Autodesk Fusion 360 part; units mm, degrees
(part 5 of 5)
sketch "Sketch13" plane through (0, 0, 4.8) normal (0, 0, 1) x (-1, 0, 0)
  circle A0 centre (1.7941, 104.2) radius 6.1
  arc A1 (-97.4773, 89.7465) -> (-97.2023, 84.7376) centre (-94.9024, 87.3758) ccw
  line L0 (-97.2023, 84.7376) -> (-47.1809, 41.1307)
  arc A2 (-48.1666, 38.5) -> (-47.1809, 41.1307) centre (-48.1666, 40) ccw
  line L1 (-48.1666, 38.5) -> (-100, 38.5)
  arc A3 (-100, 38.5) -> (-103, 35.5) centre (-100, 35.5) ccw
  line L2 (-103, 35.5) -> (-103, 28.5)
  arc A4 (-103, 28.5) -> (-100, 25.5) centre (-100, 28.5) ccw
  line L3 (-100, 25.5) -> (-42.1213, 25.5)
  arc A5 (-40, 23.3787) -> (-42.1213, 25.5) centre (-41.0607, 24.4393) ccw
  line L4 (-40, 23.3787) -> (-40, 20.8)
  arc A6 (-40, 20.8) -> (-37.5, 18.3) centre (-37.5, 20.8) ccw
  line L5 (-37.5, 18.3) -> (-34.1213, 18.3)
  arc A7 (-32, 16.1787) -> (-34.1213, 18.3) centre (-33.0607, 17.2393) ccw
  line L6 (-32, 16.1787) -> (-32, -16.1787)
  arc A8 (-34.1213, -18.3) -> (-32, -16.1787) centre (-33.0607, -17.2393) ccw
  line L7 (-34.1213, -18.3) -> (-37.5, -18.3)
  arc A9 (-37.5, -18.3) -> (-40, -20.8) centre (-37.5, -20.8) ccw
  line L8 (-40, -20.8) -> (-40, -23.3787)
  arc A10 (-42.1213, -25.5) -> (-40, -23.3787) centre (-41.0607, -24.4393) ccw
  line L9 (-42.1213, -25.5) -> (-100, -25.5)
  arc A11 (-100, -25.5) -> (-103, -28.5) centre (-100, -28.5) ccw
  line L10 (-103, -28.5) -> (-103, -35.5)
  arc A12 (-103, -35.5) -> (-100, -38.5) centre (-100, -35.5) ccw
  line L11 (-100, -38.5) -> (-48.1666, -38.5)
  arc A13 (-47.1809, -41.1307) -> (-48.1666, -38.5) centre (-48.1666, -40) ccw
  line L12 (-47.1809, -41.1307) -> (-97.2023, -84.7376)
  arc A14 (-97.2023, -84.7376) -> (-97.4773, -89.7465) centre (-94.9024, -87.3758) ccw
  arc A15 (-97.4773, -89.7465) -> (-89.0244, -98.1371) centre (0, 0) ccw
  arc A16 (-89.0244, -98.1371) -> (-85.1797, -97.5355) centre (-87.3447, -96.2855) ccw
  line L13 (-85.1797, -97.5355) -> (-74.6084, -79.2255)
  arc A17 (-71.7106, -78.449) -> (-74.6084, -79.2255) centre (-73.1595, -78.8372) ccw
  line L14 (-71.7106, -78.449) -> (-32.0836, -101.3277)
  arc A18 (-31.3071, -104.2255) -> (-32.0836, -101.3277) centre (-31.6953, -102.7766) ccw
  line L15 (-31.3071, -104.2255) -> (-41.8784, -122.5355)
  arc A19 (-41.8784, -122.5355) -> (-40.477, -126.166) centre (-39.7133, -123.7855) ccw
  arc A20 (-40.477, -126.166) -> (129.5015, -28.0288) centre (0, 0) ccw
  arc A21 (129.5015, -28.0288) -> (127.0581, -25) centre (127.0581, -27.5) ccw
  line L16 (127.0581, -25) -> (105.9155, -25)
  arc A22 (103.7941, -22.8787) -> (105.9155, -25) centre (104.8548, -23.9393) ccw
  line L17 (103.7941, -22.8787) -> (103.7941, 22.8787)
  arc A23 (105.9155, 25) -> (103.7941, 22.8787) centre (104.8548, 23.9393) ccw
  line L18 (105.9155, 25) -> (127.0581, 25)
  arc A24 (127.0581, 25) -> (129.5015, 28.0288) centre (127.0581, 27.5) ccw
  arc A25 (129.5015, 28.0288) -> (-40.477, 126.166) centre (0, 0) ccw
  arc A26 (-40.477, 126.166) -> (-41.8784, 122.5355) centre (-39.7133, 123.7855) ccw
  line L19 (-41.8784, 122.5355) -> (-31.3071, 104.2255)
  arc A27 (-32.0836, 101.3277) -> (-31.3071, 104.2255) centre (-31.6953, 102.7766) ccw
  line L20 (-32.0836, 101.3277) -> (-71.7106, 78.449)
  arc A28 (-74.6084, 79.2255) -> (-71.7106, 78.449) centre (-73.1595, 78.8372) ccw
  line L21 (-74.6084, 79.2255) -> (-85.1797, 97.5355)
  arc A29 (-85.1797, 97.5355) -> (-89.0244, 98.1371) centre (-87.3447, 96.2855) ccw
  arc A30 (-89.0244, 98.1371) -> (-97.4773, 89.7465) centre (0, 0) ccw
  circle A31 centre (-28.2185, 125.8758) radius 1.5
  arc A32 (-52.8202, -75.7299) -> (-55.718, -76.5064) centre (-54.2691, -76.1181) ccw
  line L22 (-52.8202, -75.7299) -> (-39.1739, -83.6086)
  arc A33 (-38.3975, -86.5064) -> (-39.1739, -83.6086) centre (-38.7857, -85.0575) ccw
  line L23 (-38.3975, -86.5064) -> (-38.6762, -86.9891)
  arc A34 (-41.5739, -87.7655) -> (-38.6762, -86.9891) centre (-40.125, -87.3773) ccw
  line L24 (-41.5739, -87.7655) -> (-55.2202, -79.8868)
  arc A35 (-55.9967, -76.9891) -> (-55.2202, -79.8868) centre (-55.6084, -78.438) ccw
  line L25 (-55.9967, -76.9891) -> (-55.718, -76.5064)
  circle A36 centre (123.1209, -38.5) radius 1.5
  arc A37 (-11.2762, 39.5309) -> (-14.1739, 40.3073) centre (-12.725, 39.9191) ccw
  line L26 (-11.2762, 39.5309) -> (-10.9975, 39.0482)
  arc A38 (-11.7739, 36.1504) -> (-10.9975, 39.0482) centre (-11.3857, 37.5993) ccw
  line L27 (-11.7739, 36.1504) -> (-25.4202, 28.2717)
  arc A39 (-28.318, 29.0482) -> (-25.4202, 28.2717) centre (-26.8691, 28.66) ccw
  line L28 (-28.318, 29.0482) -> (-28.5967, 29.5309)
  arc A40 (-27.8202, 32.4286) -> (-28.5967, 29.5309) centre (-28.2084, 30.9798) ccw
  line L29 (-27.8202, 32.4286) -> (-14.1739, 40.3073)
  arc A41 (-10.9975, -39.0482) -> (-11.7739, -36.1504) centre (-11.3857, -37.5993) ccw
  line L30 (-10.9975, -39.0482) -> (-11.2762, -39.5309)
  arc A42 (-14.1739, -40.3073) -> (-11.2762, -39.5309) centre (-12.725, -39.9191) ccw
  line L31 (-14.1739, -40.3073) -> (-27.8202, -32.4286)
  arc A43 (-28.5967, -29.5309) -> (-27.8202, -32.4286) centre (-28.2084, -30.9798) ccw
  line L32 (-28.5967, -29.5309) -> (-28.318, -29.0482)
  arc A44 (-25.4202, -28.2717) -> (-28.318, -29.0482) centre (-26.8691, -28.66) ccw
  line L33 (-25.4202, -28.2717) -> (-11.7739, -36.1504)
  circle A45 centre (64.5, -111.7173) radius 1.5
  arc A46 (39.8728, -10) -> (41.9941, -7.8787) centre (40.9335, -8.9393) ccw
  line L34 (39.8728, -10) -> (39.3155, -10)
  arc A47 (37.1941, -7.8787) -> (39.3155, -10) centre (38.2548, -8.9393) ccw
  line L35 (37.1941, -7.8787) -> (37.1941, 7.8787)
  arc A48 (39.3155, 10) -> (37.1941, 7.8787) centre (38.2548, 8.9393) ccw
  line L36 (39.3155, 10) -> (39.8728, 10)
  arc A49 (41.9941, 7.8787) -> (39.8728, 10) centre (40.9335, 8.9393) ccw
  line L37 (41.9941, 7.8787) -> (41.9941, -7.8787)
  circle A50 centre (-94.9024, -87.3758) radius 1.5
  circle A51 centre (-28.2185, -125.8758) radius 1.5
  circle A52 centre (64.5, 111.7173) radius 1.5
  arc A53 (-55.2202, 79.8868) -> (-55.9967, 76.9891) centre (-55.6084, 78.438) ccw
  line L38 (-55.2202, 79.8868) -> (-41.5739, 87.7655)
  arc A54 (-38.6762, 86.9891) -> (-41.5739, 87.7655) centre (-40.125, 87.3773) ccw
  line L39 (-38.6762, 86.9891) -> (-38.3975, 86.5064)
  arc A55 (-39.1739, 83.6086) -> (-38.3975, 86.5064) centre (-38.7857, 85.0575) ccw
  line L40 (-39.1739, 83.6086) -> (-52.8202, 75.7299)
  arc A56 (-55.718, 76.5064) -> (-52.8202, 75.7299) centre (-54.2691, 76.1181) ccw
  line L41 (-55.718, 76.5064) -> (-55.9967, 76.9891)
  circle A57 centre (123.1209, 38.5) radius 1.5
  circle A58 centre (45.4941, 42.5) radius 1.5
  circle A59 centre (-94.9024, 87.3758) radius 1.5
  arc A60 (94.6728, -10) -> (96.7941, -7.8787) centre (95.7335, -8.9393) ccw
  line L42 (94.6728, -10) -> (94.1155, -10)
  arc A61 (91.9941, -7.8787) -> (94.1155, -10) centre (93.0548, -8.9393) ccw
  line L43 (91.9941, -7.8787) -> (91.9941, 7.8787)
  arc A62 (94.1155, 10) -> (91.9941, 7.8787) centre (93.0548, 8.9393) ccw
  line L44 (94.1155, 10) -> (94.6728, 10)
  arc A63 (96.7941, 7.8787) -> (94.6728, 10) centre (95.7335, 8.9393) ccw
  line L45 (96.7941, 7.8787) -> (96.7941, -7.8787)
  circle A64 centre (45.4941, -42.5) radius 1.5
  line L46 (15.4941, -97) -> (41.8941, -97)
  arc A65 (45.5941, -100.7) -> (41.8941, -97) centre (41.8941, -100.7) ccw
  line L47 (45.5941, -100.7) -> (45.5941, -107.7)
  arc A66 (41.8941, -111.4) -> (45.5941, -107.7) centre (41.8941, -107.7) ccw
  line L48 (41.8941, -111.4) -> (15.4941, -111.4)
  arc A67 (11.7941, -107.7) -> (15.4941, -111.4) centre (15.4941, -107.7) ccw
  line L49 (11.7941, -107.7) -> (11.7941, -100.7)
  arc A68 (15.4941, -97) -> (11.7941, -100.7) centre (15.4941, -100.7) ccw
  line L50 (15.4941, 111.4) -> (41.8941, 111.4)
  arc A69 (45.5941, 107.7) -> (41.8941, 111.4) centre (41.8941, 107.7) ccw
  line L51 (45.5941, 107.7) -> (45.5941, 100.7)
  arc A70 (41.8941, 97) -> (45.5941, 100.7) centre (41.8941, 100.7) ccw
  line L52 (41.8941, 97) -> (15.4941, 97)
  arc A71 (11.7941, 100.7) -> (15.4941, 97) centre (15.4941, 100.7) ccw
  line L53 (11.7941, 100.7) -> (11.7941, 107.7)
  arc A72 (15.4941, 111.4) -> (11.7941, 107.7) centre (15.4941, 107.7) ccw
  circle A73 centre (97.2941, 62.4) radius 1.5
  circle A74 centre (97.2941, -62.4) radius 1.5
  circle A75 centre (64.2941, 62.4) radius 1.5
  circle A76 centre (64.2941, -62.4) radius 1.5
  arc A77 (65.7941, -100.26) -> (68.1301, -101.5054) centre (67.2941, -100.26) ccw
  line L54 (65.7941, -100.26) -> (65.7941, -74.3)
  arc A78 (67.2941, -72.8) -> (65.7941, -74.3) centre (67.2941, -74.3) ccw
  line L55 (67.2941, -72.8) -> (95.1844, -72.8)
  arc A79 (96.3668, -75.223) -> (95.1844, -72.8) centre (95.1844, -74.3) ccw
  arc A80 (68.1301, -101.5054) -> (96.3668, -75.223) centre (0, 0) ccw
  arc A81 (65.7941, 74.3) -> (67.2941, 72.8) centre (67.2941, 74.3) ccw
  line L56 (65.7941, 74.3) -> (65.7941, 100.26)
  arc A82 (68.1301, 101.5054) -> (65.7941, 100.26) centre (67.2941, 100.26) ccw
  arc A83 (96.3668, 75.223) -> (68.1301, 101.5054) centre (0, 0) ccw
  arc A84 (95.1844, 72.8) -> (96.3668, 75.223) centre (95.1844, 74.3) ccw
  line L57 (95.1844, 72.8) -> (67.2941, 72.8)
  circle A85 centre (0, 0) radius 3
  circle A86 centre (-100, 35.5) radius 1.5
  circle A87 centre (-53.2894, -35.5) radius 1.5
  circle A88 centre (-53.2894, 35.5) radius 1.5
  circle A89 centre (-100, -35.5) radius 1.5
  line L58 (13.9155, 56) -> (55.6728, 56)
  line L59 (57.7941, 58.1213) -> (57.7941, 83.8787)
  line L60 (55.6728, -56) -> (13.9155, -56)
  line L61 (57.7941, -58.1213) -> (57.7941, -83.8787)
  line L62 (56.2941, -56) -> (22.2941, -56)
  line L63 (20.7941, -57.5) -> (20.7941, -90.5)
  line L64 (22.2941, -92) -> (56.2941, -92)
  line L65 (57.7941, -90.5) -> (57.7941, -57.5)
  arc A90 (56.2941, -92) -> (57.7941, -90.5) centre (56.2941, -90.5) ccw
  arc A91 (20.7941, -90.5) -> (22.2941, -92) centre (22.2941, -90.5) ccw
  arc A92 (57.7941, -57.5) -> (56.2941, -56) centre (56.2941, -57.5) ccw
  arc A93 (22.2941, -56) -> (20.7941, -57.5) centre (22.2941, -57.5) ccw
  line L66 (56.2941, 56) -> (22.2941, 56)
  line L67 (20.7941, 57.5) -> (20.7941, 90.5)
  line L68 (22.2941, 92) -> (56.2941, 92)
  line L69 (57.7941, 90.5) -> (57.7941, 57.5)
  arc A94 (56.2941, 56) -> (57.7941, 57.5) centre (56.2941, 57.5) ccw
  arc A95 (20.7941, 57.5) -> (22.2941, 56) centre (22.2941, 57.5) ccw
  arc A96 (57.7941, 90.5) -> (56.2941, 92) centre (56.2941, 90.5) ccw
  arc A97 (22.2941, 92) -> (20.7941, 90.5) centre (22.2941, 90.5) ccw
  point P0 (57.7941, -56)
  point P1 (20.7941, -56)
  point P2 (57.7941, -92)
  point P3 (57.7941, 56)
  point P4 (20.7941, 56)
  point P5 (57.7941, 92)
  dimension "d405" = 37
  dimension "d406" = 36
  dimension "d407" = 1.5
  dimension "d408" = 1.5
  dimension "d409" = 1.5
  dimension "d410" = 1.5
  dimension "d411" = 37
  dimension "d412" = 36
  dimension "d413" = 1.5
  dimension "d414" = 1.5
  dimension "d415" = 1.5
  dimension "d416" = 1.5
  constraint horizontal L62
  constraint vertical L63
  constraint horizontal L64
  constraint vertical L65
  constraint collinear L61 L65
  constraint collinear L60 L62
  constraint coincident P2 L65
  constraint coincident P2 L64
  constraint tangent L65 A90
  constraint tangent L64 A90
  constraint tangent L64 A91
  constraint tangent L63 A91
  constraint coincident P0 L65
  constraint coincident P0 L62
  constraint tangent L65 A92
  constraint tangent L62 A92
  constraint coincident P1 L62
  constraint coincident P1 L63
  constraint tangent L62 A93
  constraint tangent L63 A93
  constraint horizontal L66
  constraint vertical L67
  constraint horizontal L68
  constraint vertical L69
  constraint collinear L58 L66
  constraint collinear L59 L69
  constraint coincident P3 L69
  constraint coincident P3 L66
  constraint tangent L69 A94
  constraint tangent L66 A94
  constraint coincident P4 L66
  constraint coincident P4 L67
  constraint tangent L66 A95
  constraint tangent L67 A95
  constraint coincident P5 L69
  constraint coincident P5 L68
  constraint tangent L69 A96
  constraint tangent L68 A96
  constraint tangent L68 A97
  constraint tangent L67 A97
  measures "d405" distance of P0 P1
  measures "d406" distance of P0 P2
  measures "d407" radius of A90
  measures "d408" radius of A91
  measures "d409" radius of A92
  measures "d410" radius of A93
  measures "d411" distance of P3 P4
  measures "d412" distance of P3 P5
  measures "d413" radius of A94
  measures "d414" radius of A95
  measures "d415" radius of A96
  measures "d416" radius of A97
extrude "Extrude17" cut sketch "Sketch13" against normal through all contours L58 L59 L66 L67 L68 L69 A94 A95 A96 A97 | L60 L61 L62 L63 L64 L65 A90 A91 A92 A93
